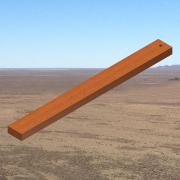
# Autodesk Inventor part: splashFurring
Saved by Autodesk Inventor 2014 SP1 (Build 180222100, 222)
## iProperties
Created: 2014-05-01
Part Number: splashFurring
Material: Wood (Cherry)
Document SubType Name: Modeling
Designer: Dave
Mass: 362.367 g
Surface Area: 1011.29 cm^2
Volume: 575.186 cm^3
Density: 0.63 g/cm^3
Appearance: Cherry - Natural Low Gloss
Author: Dave
Autodesk Inventor part; units mm, degrees
ref_plane "YZ Plane" through (0, 0, 0) normal (1, 0, 0) x (0, 1, 0)
ref_plane "XZ Plane" through (0, 0, 0) normal (0, 1, 0) x (-1, 0, 0)
ref_plane "XY Plane" through (0, 0, 0) normal (0, 0, 1) x (1, 0, 0)
sketch "Sketch1" plane through (0, 0, 0) normal (0, 0, 1) x (1, 0, 0)
  line L0 (0, 0) -> (38.1, 0)
  line L1 (38.1, 0) -> (38.1, 16.51)
  line L2 (38.1, 16.51) -> (0, 16.51)
  line L3 (0, 16.51) -> (0, 0)
  dimension "d0" = 38.1
  dimension "d1" = 16.51
  constraints: 8 end point, 2 parallel, 1 horizontal, 1 perpendicular
  measures "d0" distance of L0.start L0.end
  measures "d1" distance of L2.end L0.start
extrude "Extrusion1" add sketch "Sketch1" along normal blind 406.4
sketch "Sketch3" plane through (0, 16.51, 0) normal (0, 1, 0) x (1, 0, 0)
  circle A0 centre (19.05, -12.7) radius 3.175
  line L0 (38.1, 0) -> (0, 0) projected
  dimension "d11" = 6.35
  dimension "d19" = 12.7
  constraints: 1 centre point
  measures "d11" diameter of A0
  measures "d19" distance from line of A0.centre L0
hole "Hole2" at (19.05, 16.51, 12.7) direction (0, -1, 0) diameter 6.35 end through all
body "Solid1"
